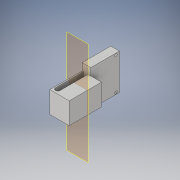
# Autodesk Inventor part: kinect_fixt
Saved by Autodesk Inventor 2019 (Build 230136000, 136)
## iProperties
Created: 2024-05-02
Part Number: kinect_fixt
Material: Generisch
Document SubType Name: Modeling
Designer: nic
Density: 1 g/cm^3
Appearance: Vorgabe
Author: nic
Autodesk Inventor part; units mm, degrees
ref_plane "YZ Plane" through (0, 0, 0) normal (1, 0, 0) x (0, 1, 0)
ref_plane "XZ Plane" through (0, 0, 0) normal (0, 1, 0) x (-1, 0, 0)
ref_plane "XY Plane" through (0, 0, 0) normal (0, 0, 1) x (1, 0, 0)
ref_plane "Arbeitsebene1" through (0, 0, 0) normal (0, 0, 1) x (1, 0, 0)
sketch "Skizze1" plane through (0, 0, 0) normal (0, 0, 1) x (1, 0, 0)
  circle A0 centre (-13.5, 65) radius 3 construction
  circle A1 centre (-13.5, 65) radius 3 construction
  line L0 (0, 130) -> (0, 0) construction
  line L1 (0, 130) -> (-27, 130) construction
  line L2 (-27, 0) -> (-27, 130) construction
  line L3 (0, 0) -> (-27, 0) construction
  line L4 (-27, 80) -> (0, 80)
  line L5 (0, 80) -> (0, 50)
  line L6 (0, 50) -> (-27, 50)
  line L7 (-27, 50) -> (-27, 80)
  line L8 (-27, 80) -> (0, 50) construction
  line L9 (0, 80) -> (-27, 50) construction
  dimension "d0" = 30
  constraints: 12 end point, 2 midpoint, 2 parallel, 1 horizontal, 1 perpendicular, 1 point on line
  measures "d0" distance of L4.end L5.end
extrude "Extrusion1" add sketch "Skizze1" along normal blind 25
sketch "Skizze3" plane through (-27, 80, 0) normal (0, 1, 0) x (1, 0, 0)
  line L0 (0, 0) -> (0, -25) projected
  line L1 (0, 0) -> (5.0639, 0)
  line L2 (5.0639, 0) -> (5.0639, -24.302)
  line L3 (5.0639, -24.302) -> (0, -24.302)
  line L4 (0, -24.302) -> (0, 0)
  circle A0 centre (5.0639, -18.8642) radius 3.15
  circle A1 centre (5.0639, -8.0952) radius 3.15
  circle A2 centre (5.0639, -12.5) radius 3.25
  point P0 (27, 0)
  dimension "d6" = 6.3
  dimension "d7" = 6.3
  dimension "d10" = 6.5
  constraints: 8 end point, 3 centre point, 3 point on line, 2 parallel, 1 horizontal, 1 perpendicular
  measures "d6" diameter of A0
  measures "d7" diameter of A1
  measures "d10" diameter of A2
extrude "Extrusion4" cut sketch "Skizze3" against normal through all contours A2 A1 L2 | L2 A1 A2 | A1 L2 A0 A2 | A2 A0 L2 | L2 A0 A2 | A1 A2 A0 L2 picked at (5.2798, -10.5577) picked at (4.848, -10.5577) picked at (5.0263, -15.7268) picked at (5.1015, -15.7268)
sketch "Skizze5" plane through (-27, 50, 0) normal (0, -1, 0) x (1, 0, 0)
  circle A0 centre (5.0639, 12.5) radius 3.25 construction
  line L0 (5.0639, 18.9193) -> (5.0639, 6.0807) construction
  line L1 (1.812, 18.9193) -> (1.812, 6.0807)
  line L2 (8.3158, 6.0807) -> (8.3158, 18.9193)
  arc A1 (8.3158, 18.9193) -> (1.812, 18.9193) centre (5.0639, 18.9193) ccw
  arc A2 (1.812, 6.0807) -> (8.3158, 6.0807) centre (5.0639, 6.0807) ccw
  point P0 (27, 0)
  constraints: 8 end point, 4 point on circle, 4 tangent, 2 centre point, 1 midpoint, 1 parallel, 1 vertical
extrude "Extrusion6" cut sketch "Skizze5" against normal through all
sketch "Skizze6" plane through (0, 0, 0) normal (0, 0, -1) x (-1, 0, 0)
  line L0 (27, 50) -> (0, 50) projected
  line L1 (27, 80) -> (0, 80) projected
  line L2 (27, 50) -> (15, 50)
  line L3 (15, 50) -> (15, 80)
  line L4 (15, 80) -> (27, 80)
  line L5 (27, 80) -> (27, 50)
  point P0 (0, 0)
  dimension "d20" = 12
  constraints: 8 end point, 2 parallel, 1 horizontal, 1 perpendicular, 1 point on line
  measures "d20" distance of L3.end L4.end
extrude "Extrusion7" add sketch "Skizze6" along normal blind 60
sketch "Skizze7" plane through (-27, 80, 25) normal (0, 1, 0) x (1, 0, 0)
  line L0 (12, 25) -> (27, 25) construction
  line L1 (12, 25) -> (12, 85) construction
  line L2 (0, 85) -> (12, 85) construction
  line L3 (0, 85) -> (0, 0) construction
  line L4 (27, 0) -> (0, 0) construction
  line L5 (27, 25) -> (27, 0) construction
  arc A0 (8.3158, 18.9193) -> (1.812, 18.9193) centre (5.0639, 18.9193) ccw construction
  line L6 (8.3158, 18.9193) -> (8.3158, 6.0807) construction
  arc A1 (1.812, 6.0807) -> (8.3158, 6.0807) centre (5.0639, 6.0807) ccw construction
  line L7 (1.812, 6.0807) -> (1.812, 18.9193) construction
  line L8 (5.0639, 18.9193) -> (5.0639, 77.8219) construction
  line L9 (8.3158, 18.9193) -> (8.3158, 77.8219)
  line L10 (1.812, 77.8219) -> (1.812, 18.9193)
  arc A2 (1.812, 18.9193) -> (8.3158, 18.9193) centre (5.0639, 18.9193) ccw
  arc A3 (8.3158, 77.8219) -> (1.812, 77.8219) centre (5.0639, 77.8219) ccw
  point P0 (27, 25)
  point P1 (5.0639, 48.3706)
  constraints: 8 end point, 4 point on circle, 4 tangent, 2 centre point, 2 parallel, 1 midpoint
extrude "Extrusion8" cut sketch "Skizze7" against normal through all
sketch "Skizze8" plane through (0, 0, 0) normal (0, 0, -1) x (-1, 0, 0)
  line L0 (15, 50) -> (15, 80) projected
  line L1 (15, 80) -> (0, 80) projected
  line L2 (0, 80) -> (0, 50) projected
  line L3 (0, 50) -> (15, 50) projected
  point P0 (0, 0)
extrude "Extrusion9" add sketch "Skizze8" along normal blind 20
sketch "Skizze10" plane through (-27, 50, 25) normal (0, -1, 0) x (1, 0, 0)
  line L0 (1.812, -77.8219) -> (1.812, -6.0807) projected
  arc A0 (8.3158, -6.0807) -> (1.812, -6.0807) centre (5.0639, -6.0807) ccw projected
  line L1 (8.3158, -6.0807) -> (8.3158, -77.8219) projected
  arc A1 (1.812, -77.8219) -> (8.3158, -77.8219) centre (5.0639, -77.8219) ccw projected
  line L2 (27, 0) -> (27, -45) projected
  line L3 (0, 0) -> (27, 0) projected
  line L4 (0, 0) -> (0, -85) projected
  line L5 (12, -85) -> (0, -85) projected
  line L6 (12, -45) -> (12, -85) projected
  line L7 (27, -45) -> (12, -45) projected
  line L8 (12, -45) -> (12, -85) projected
  line L9 (12, -45) -> (0, -45)
  point P0 (27, -25)
  constraints: 2 end point, 1 perpendicular, 1 point on line
extrude "Extrusion10" add sketch "Skizze10" along normal blind 10 contours A1 L1 L9 L6 L5 L4 L0 | L0 L9 L1 A1
sketch "Skizze11" plane through (-27, 80, 25) normal (0, 1, 0) x (1, 0, 0)
  line L0 (0, 85) -> (0, 0) projected
  line L1 (27, 0) -> (0, 0) projected
  line L2 (27, 0) -> (27, 45) projected
  line L3 (12, 45) -> (27, 45) projected
  line L4 (12, 45) -> (12, 85) projected
  line L5 (0, 85) -> (12, 85) projected
  line L6 (1.812, 6.0807) -> (1.812, 77.8219) projected
  arc A0 (8.3158, 77.8219) -> (1.812, 77.8219) centre (5.0639, 77.8219) ccw projected
  line L7 (8.3158, 77.8219) -> (8.3158, 6.0807) projected
  arc A1 (1.812, 6.0807) -> (8.3158, 6.0807) centre (5.0639, 6.0807) ccw projected
  line L8 (12, 45) -> (0, 45) projected
  line L9 (12, 45) -> (0, 45)
  point P0 (27, 25)
  constraints: 2 end point, 1 perpendicular
extrude "Extrusion11" add sketch "Skizze11" along normal blind 10 contours L5 L4 L8 L7 A0 L6 L0 | L6 A0 L7 L8
sketch "Skizze13" plane through (-27, 40, 25) normal (0, -1, 0) x (1, 0, 0)
  line L0 (0, -85) -> (12, -85) projected
  line L1 (12, -85) -> (12, -45) projected
  line L2 (12, -45) -> (0, -45) projected
  line L3 (0, -45) -> (0, -85) projected
  point P0 (27, -25)
extrude "Extrusion12" add sketch "Skizze13" against normal up to surface (50 mm away)
sketch "Skizze14" plane through (-27, 50, 25) normal (-1, 0, 0) x (0, 0, 1)
  line L0 (-85, 40) -> (-85, -10) projected
  line L1 (-85, 15) -> (-0.0726, 15)
  line L2 (-85, 21.5305) -> (-80, 21.5305)
  line L3 (-80, 15) -> (-80, 37.5)
  line L4 (-80, 37.5) -> (-80, -7.5)
  circle A0 centre (-80, -7.5) radius 1.75
  circle A1 centre (-80, 37.5) radius 1.75
  point P0 (-25, -50)
  dimension "d38" = 5
  dimension "d39" = 22.5
  dimension "d40" = 45
  dimension "d41" = 3.5
  dimension "d42" = 3.5
  constraints: 8 end point, 4 coincident, 3 point on line, 2 centre point, 1 horizontal, 1 midpoint, 1 perpendicular, 1 vertical
  measures "d38" distance of L2.start L2.end
  measures "d39" distance of L3.start L3.end
  measures "d40" distance of L3.end L4.end
  measures "d41" diameter of A0
  measures "d42" diameter of A1
extrude "Extrusion13" cut sketch "Skizze14" against normal through all contours A1 | A0
